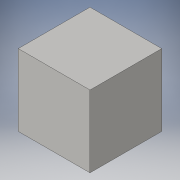
# Autodesk Inventor part: WoodenBlock
Saved by Autodesk Inventor 2016 (Build 200138000, 138)
## iProperties
Created: 2017-03-02
Part Number: WoodenBlock
Material: Generic
Document SubType Name: Modeling
Designer: fhs-mgr
Density: 1 g/cm^3
Appearance: Default
Author: fhs-mgr
Autodesk Inventor part; units mm, degrees
ref_plane "YZ Plane" through (0, 0, 0) normal (1, 0, 0) x (0, 1, 0)
ref_plane "XZ Plane" through (0, 0, 0) normal (0, 1, 0) x (-1, 0, 0)
ref_plane "XY Plane" through (0, 0, 0) normal (0, 0, 1) x (1, 0, 0)
sketch "Sketch1" plane through (0, 0, 0) normal (0, 1, 0) x (-1, 0, 0)
  line L0 (0, 0) -> (19.05, 0)
  line L1 (19.05, 0) -> (19.05, -19.05)
  line L2 (19.05, -19.05) -> (0, -19.05)
  line L3 (0, -19.05) -> (0, 0)
  dimension "d0" = 19.05
  dimension "d1" = 19.05
  constraints: 8 end point, 2 parallel, 1 horizontal, 1 perpendicular
  measures "d0" distance of L1.end L2.end
  measures "d1" distance of L0.end L1.end
extrude "Extrusion1" add sketch "Sketch1" along normal blind 19.05
body "Solid1"
